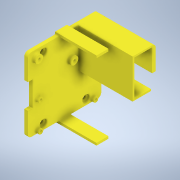
# Autodesk Inventor part: pieza_nasa
Saved by Autodesk Inventor 2021 (Build 250183000, 183)
## iProperties
Created: 2024-10-05
Part Number: pieza_nasa
Material: Generic
Document SubType Name: Modeling
Designer: hojan
Density: 1 g/cm^3
Appearance: Default
Author: hojan
Autodesk Inventor part; units mm, degrees
ref_plane "YZ Plane" through (0, 0, 0) normal (1, 0, 0) x (0, 1, 0)
ref_plane "XZ Plane" through (0, 0, 0) normal (0, 1, 0) x (-1, 0, 0)
ref_plane "XY Plane" through (0, 0, 0) normal (0, 0, 1) x (1, 0, 0)
sketch "Boceto1" plane through (0, 0, 0) normal (1, 0, 0) x (0, 1, 0)
  line L0 (-31, 31) -> (31, 31)
  line L1 (31, 31) -> (31, -31)
  line L2 (31, -31) -> (-31, -31)
  line L3 (-31, -31) -> (-31, 31)
  line L4 (-31, 31) -> (31, -31) construction
  line L5 (31, 31) -> (-31, -31) construction
  point P0 (0, 0)
  dimension "d0" = 62
  dimension "d1" = 62
  constraints: 12 end point, 2 midpoint, 2 parallel, 1 horizontal, 1 perpendicular
  measures "d0" distance of L1.end L2.end
  measures "d1" distance of L0.end L1.end
extrude "Extrusión1" add sketch "Boceto1" along normal blind 3
sketch "Boceto2" plane through (3, 0, 0) normal (1, 0, 0) x (0, 0, -1)
  line L0 (0, 0) -> (18, 0)
  line L1 (18, 0) -> (18, 26)
  line L2 (18, 26) -> (-18, 26)
  line L3 (-18, 26) -> (-18, -26)
  line L4 (-18, -26) -> (18, -26)
  circle A0 centre (-18, 26) radius 1.5
  circle A1 centre (18, 26) radius 1.5
  circle A2 centre (-18, -26) radius 1.5
  circle A3 centre (18, -26) radius 1.5
  dimension "d4" = 18
  dimension "d5" = 26
  dimension "d6" = 36
  dimension "d7" = 52
  dimension "d8" = 3
  dimension "d9" = 3
  dimension "d10" = 3
  dimension "d11" = 3
  constraints: 10 end point, 4 centre point, 4 coincident, 3 perpendicular, 1 horizontal, 1 point on line, 1 vertical
  measures "d4" distance of L0.start L0.end
  measures "d5" distance of L0.end L1.end
  measures "d6" distance of L1.end L2.end
  measures "d7" distance of L2.end L3.end
  measures "d8" diameter of A0
  measures "d9" diameter of A1
  measures "d10" diameter of A2
  measures "d11" diameter of A3
extrude "Extrusión2" cut sketch "Boceto2" against normal blind 3
fillet "Empalme1" radius 3 4 edges at (1.5, 31, 31) (1.5, 31, -31) (1.5, -31, 31) (1.5, -31, -31)
sketch "Boceto3" plane through (3, 0, 0) normal (1, 0, 0) x (0, 0, -1)
  circle A0 centre (-18, 26) radius 1.5 projected
  circle A1 centre (-18, 26) radius 3
  circle A2 centre (18, 26) radius 1.5 projected
  circle A3 centre (18, 26) radius 3
  circle A4 centre (18, -26) radius 1.5 projected
  circle A5 centre (18, -26) radius 3
  circle A6 centre (-18, -26) radius 1.5 projected
  circle A7 centre (-18, -26) radius 3
  point P0 (0, 0)
  dimension "d15" = 6
  dimension "d16" = 6
  dimension "d17" = 6
  dimension "d18" = 6
  constraints: 4 centre point, 4 coincident
  measures "d15" diameter of A1
  measures "d16" diameter of A3
  measures "d17" diameter of A5
  measures "d18" diameter of A7
extrude "Extrusión3" cut sketch "Boceto3" against normal blind 1.5 contours A0 | A1 | A2 | A3 | A5 | A7
sketch "Boceto4" plane through (3, 0, 0) normal (1, 0, 0) x (0, 0, -1)
  line L0 (0, 0) -> (-27, 0)
  line L1 (0, 0) -> (-31, 0)
  line L2 (-31, 28) -> (-31, -28) projected
  line L3 (-27, 0) -> (-27, 10.5)
  line L4 (-27, 10.5) -> (-31, 10.5)
  line L5 (-31, 10.5) -> (-31, -10.5)
  line L6 (-31, -10.5) -> (-27, -10.5)
  line L7 (-27, -10.5) -> (-27, 0)
  line L8 (0, 12.3803) -> (0, 8.7582)
  line L9 (27, 0) -> (27, 10.5)
  line L10 (27, 10.5) -> (31, 10.5)
  line L11 (31, 10.5) -> (31, -10.5)
  line L12 (31, -10.5) -> (27, -10.5)
  line L13 (27, -10.5) -> (27, 0)
  point P0 (31, 0)
  dimension "d21" = 27
  dimension "d22" = 31
  dimension "d23" = 10.5
  dimension "d24" = 21
  constraints: 26 end point, 6 symmetric about line, 5 perpendicular, 2 point on line, 2 vertical, 1 horizontal
  measures "d21" distance of L0.start L0.end
  measures "d22" distance of L0.start L1.end
  measures "d23" distance of L0.end L3.end
  measures "d24" distance of L4.end L5.end
extrude "Extrusión4" cut sketch "Boceto4" against normal blind 3
sketch "Boceto5" plane through (3, 0, 0) normal (1, 0, 0) x (0, 0, -1)
  arc A0 (-28, 31) -> (-31, 28) centre (-28, 28) ccw projected
  line L0 (-28, 28) -> (15, 28)
  line L1 (15, 28) -> (15, 7)
  line L2 (15, 7) -> (-28, 7)
  line L3 (-28, 28) -> (-28, 25.46)
  line L4 (-28, 25.46) -> (-21.4, 25.46)
  line L5 (15, 7) -> (15, 9.5)
  line L6 (15, 9.5) -> (8.4, 9.5)
  circle A1 centre (-21.4, 25.46) radius 1
  circle A2 centre (8.4, 9.5) radius 1
  circle A3 centre (-21.4, 25.46) radius 3.25
  circle A4 centre (8.4, 9.5) radius 3.25
  circle A5 centre (-18, 26) radius 1.5 projected
  circle A6 centre (-18, 26) radius 3 projected
  line L7 (-28, 28) -> (-31, 28)
  line L8 (-31, 28) -> (12, 28)
  line L9 (12, 7) -> (-31, 7)
  circle A7 centre (5.4, 9.5) radius 1
  line L10 (12, 28) -> (12, 7)
  circle A8 centre (5.4, 9.5) radius 3.25
  line L11 (12, 9.5) -> (5.4, 9.5)
  line L12 (12, 7) -> (12, 9.5)
  circle A9 centre (-24.4, 25.46) radius 1
  line L13 (-31, 25.46) -> (-24.4, 25.46)
  line L14 (-31, 28) -> (-31, 25.46)
  line L15 (-31, 28) -> (-34, 28)
  circle A10 centre (-24.4, 25.46) radius 3.25
  point P0 (0, 0)
  point P1 (-19.0678, 23.1965)
  point P2 (-19.8839, 28.3347)
  point P3 (-21, 26)
  point P4 (-21, 26)
  point P5 (-31, 31)
  dimension "d27" = 43
  dimension "d28" = 21
  dimension "d29" = 2.54
  dimension "d30" = 6.6
  dimension "d31" = 2.5
  dimension "d32" = 6.6
  dimension "d33" = 2
  dimension "d34" = 2
  dimension "d35" = 6.5
  dimension "d36" = 6.5
  dimension "d65" = 3
  dimension "d68" = 3
  constraints: 32 end point, 8 centre point, 8 coincident, 4 horizontal, 3 perpendicular, 2 point on line, 1 collinear, 1 vertical, 27 other
  measures "d27" distance of L0.start L0.end
  measures "d28" distance of L0.end L1.end
  measures "d29" distance of L0.start L3.end
  measures "d30" distance of L3.end L4.end
  measures "d31" distance of L1.end L5.end
  measures "d32" distance of L5.end L6.end
  measures "d33" diameter of A1
  measures "d34" diameter of A2
  measures "d35" diameter of A3
  measures "d36" diameter of A4
  measures "d65" distance of L0.start L7.end
  measures "d68" distance of L0.start L8.start
extrude "Extrusión5" add sketch "Boceto5" along normal blind 3 contours A10 L0 A3 | A3 L0 A10 | A8 A2 L11 A7 A4 | A4 A7 L2 A8 | A10 A1 L4 A9 A3 L0 | A10 L4 A9 A3 | A3 A9 L4 A1 A10 | A3 A9 L4 A10 L0 | A8 A2 L11 L6 | L6 L11 A2 A8 | A8 L2 A4 A7 L11 A2 | L2 A4 A8 | A8 A4 L2 | A10 A1 picked at (4.536, 6.8619) picked at (7.0312, 6.9529)
fillet "Empalme2" radius 1 2 edges at (3, 25.46, 27.65) (3, 9.5, -2.15)
sketch "Boceto6" plane through (3, 0, 0) normal (1, 0, 0) x (0, 0, -1)
  line L0 (-31, -35) -> (-31, -21.2021)
  line L1 (-31, 28) -> (-31, -28) projected
  line L2 (-31, -21.2021) -> (-23, -21.2021)
  line L3 (-23, -21.2021) -> (-23, 1.7979)
  line L4 (-23, 1.7979) -> (23.5, 1.7979)
  line L5 (23.5, 1.7979) -> (23.5, -21.2021)
  line L6 (23.5, -21.2021) -> (-23, -21.2021)
  line L7 (-1.735, -21.2021) -> (-1.735, -27.2021)
  circle A0 centre (23.5, 1.7979) radius 2
  circle A1 centre (23.5, -21.2021) radius 2
  circle A2 centre (-23, -21.2021) radius 2
  circle A3 centre (-23, 1.7979) radius 2
  circle A4 centre (-23, 1.7979) radius 1
  circle A5 centre (23.5, -21.2021) radius 1
  circle A6 centre (-23, -21.2021) radius 1
  circle A7 centre (23.5, 1.7979) radius 1
  line L8 (-23, -5.2021) -> (23.5, -5.2021)
  line L9 (23.5, -28.2021) -> (-23, -28.2021)
  line L10 (-1.735, -28.2021) -> (-1.735, -34.2021)
  circle A8 centre (-23, -5.2021) radius 1
  line L11 (-23, -28.2021) -> (-23, -5.2021)
  circle A9 centre (-23, -28.2021) radius 2
  circle A10 centre (-23, -5.2021) radius 2
  line L12 (23.5, -5.2021) -> (23.5, -28.2021)
  circle A11 centre (23.5, -28.2021) radius 1
  circle A12 centre (23.5, -5.2021) radius 1
  circle A13 centre (23.5, -28.2021) radius 2
  circle A14 centre (23.5, -5.2021) radius 2
  line L13 (-31, -28.2021) -> (-23, -28.2021)
  circle A15 centre (-23, -28.2021) radius 1
  point P0 (0, 0)
  point P1 (0, -7)
  point P2 (-31, -35)
  dimension "d40" = 23
  dimension "d41" = 46.5
  dimension "d42" = 8
  dimension "d43" = 13.7979
  dimension "d44" = 6
  dimension "d45" = 4
  dimension "d46" = 4
  dimension "d47" = 4
  dimension "d48" = 4
  dimension "d49" = 2
  dimension "d50" = 2
  dimension "d51" = 2
  dimension "d52" = 2
  dimension "d81" = 7
  constraints: 26 end point, 16 centre point, 16 coincident, 3 perpendicular, 3 point on line, 3 vertical, 1 collinear, 1 horizontal, 30 other
  measures "d40" distance of L2.end L3.end
  measures "d41" distance of L3.end L4.end
  measures "d42" distance of L0.end L2.end
  measures "d43" distance of L0.start L0.end
  measures "d44" distance of L7.start L7.end
  measures "d45" diameter of A0
  measures "d46" diameter of A1
  measures "d47" diameter of A2
  measures "d48" diameter of A3
  measures "d49" diameter of A4
  measures "d50" diameter of A5
  measures "d51" diameter of A6
  measures "d52" diameter of A7
  measures "d81" distance of point (0, 0) point (0, -7)
extrude "Extrusión6" add sketch "Boceto6" along normal up to surface (3 mm away) contours L13 A15 L9 A9 | A9 L11 A15 L13 | A9 L9 A15 L11 | A13 L12 A11 L9 | L9 A11 L12 A13 | A10 L3 A8 | L3 A8 L8 A10 | A10 L8 A8 L3 | A14 L5 A12 L8 | L8 A12 L5 A14 | A14 L5 A12
fillet "Empalme3" radius 1 4 edges at (3, -28.2021, -21.5) (3, -5.2021, -21.5) (3, -5.2021, 25) (3, -28.2021, 25)
sketch "Boceto8" plane through (3, 0, 0) normal (1, 0, 0) x (0, 0, -1)
  circle A0 centre (-23, -5.2021) radius 3 projected
  circle A1 centre (5.4, 9.5) radius 4.25 projected
  arc A2 (-20.6357, 27.4329) -> (-20.3583, 24.1457) centre (-24.4, 25.46) ccw projected
  arc A3 (-20.3583, 24.1457) -> (-20.6357, 27.4329) centre (-18, 26) ccw projected
  arc A4 (-20.9998, -25.9662) -> (-24.0825, -31) centre (-23, -28.2021) ccw projected
  arc A5 (-20.0002, -28.2359) -> (-20.9998, -25.9662) centre (-18, -26) ccw projected
  arc A6 (-21.9175, -31) -> (-20.0002, -28.2359) centre (-23, -28.2021) ccw projected
  line L0 (-21.9175, -31) -> (22.4175, -31) projected
  arc A7 (20.5736, -27.5416) -> (22.4175, -31) centre (23.5, -28.2021) ccw projected
  arc A8 (20.9264, -26.6606) -> (20.5736, -27.5416) centre (18, -26) ccw projected
  arc A9 (24.5825, -31) -> (20.9264, -26.6606) centre (23.5, -28.2021) ccw projected
  line L1 (24.5825, -31) -> (28, -31) projected
  arc A10 (28, -31) -> (31, -28) centre (28, -28) ccw projected
  line L2 (31, -28) -> (31, -10.5) projected
  line L3 (31, -10.5) -> (27, -10.5) projected
  line L4 (27, -10.5) -> (27, 10.5) projected
  line L5 (27, 10.5) -> (31, 10.5) projected
  line L6 (31, 10.5) -> (31, 28) projected
  arc A11 (31, 28) -> (28, 31) centre (28, 28) ccw projected
  line L7 (28, 31) -> (-28, 31) projected
  arc A12 (-28, 31) -> (-31, 28) centre (-28, 28) ccw projected
  line L8 (-31, 28) -> (-31, 10.5) projected
  line L9 (-31, 10.5) -> (-27, 10.5) projected
  line L10 (-27, 10.5) -> (-27, -10.5) projected
  line L11 (-27, -10.5) -> (-31, -10.5) projected
  line L12 (-31, -10.5) -> (-31, -28) projected
  arc A13 (-31, -28) -> (-28, -31) centre (-28, -28) ccw projected
  line L13 (-28, -31) -> (-24.0825, -31) projected
  circle A14 centre (18, 26) radius 3 projected
  circle A15 centre (23.5, -5.2021) radius 3 projected
  line L14 (28, 31) -> (-28, 31) projected
  line L15 (28, 31) -> (28, 29.5)
  line L16 (28, 29.5) -> (13, 29.5)
  line L17 (13, 29.5) -> (13, -0.5)
  line L18 (13, -0.5) -> (27, -0.5)
  line L19 (27, -10.5) -> (27, 10.5) projected
  line L20 (27, -0.5) -> (27, 10.5)
  line L21 (27, 10.5) -> (31, 10.5)
  line L22 (28, 29.5) -> (28, 10.5)
  line L23 (13, 29.5) -> (11.5, 29.5)
  line L24 (11.5, 29.5) -> (11.5, 31)
  line L25 (11.5, 29.5) -> (11.5, -2)
  line L26 (11.5, -2) -> (27, -2)
  line L27 (27, -2) -> (27, -0.5)
  point P0 (0, 0)
  dimension "d89" = 1.5
  dimension "d90" = 15
  dimension "d91" = 30
  dimension "d92" = 1.5
  dimension "d93" = 31.5
  constraints: 24 end point, 9 perpendicular, 5 point on line, 1 parallel, 1 vertical
  measures "d89" distance of L7.start L15.end
  measures "d90" distance of L15.end L16.end
  measures "d91" distance of L16.end L17.end
  measures "d92" distance of L16.end L23.end
  measures "d93" distance of L23.end L25.end
extrude "Extrusión8" add sketch "Boceto8" along normal blind 46 contours L7 L15 L16 L23 L24 | A11 L6 L5 L22 L15 | L23 L17 L18 L4 L26 L25
sketch "Boceto10" plane through (0, 0, 0) normal (-1, 0, 0) x (0, 0, 1)
  line L0 (28, -31) -> (-28, -31) projected
  line L1 (0, -31) -> (-5, -31)
  line L2 (-5, -31) -> (-5, -33)
  line L3 (-5, -33) -> (5, -33)
  line L4 (5, -33) -> (5, -31)
  line L5 (5, -31) -> (0, -31)
  line L6 (0, 0) -> (-3.9582, 0)
  line L7 (0, 31) -> (-5, 31)
  line L8 (-5, 31) -> (-5, 33)
  line L9 (-5, 33) -> (5, 33)
  line L10 (5, 33) -> (5, 31)
  line L11 (5, 31) -> (0, 31)
  dimension "d96" = 5
  dimension "d97" = 2
  dimension "d98" = 10
  constraints: 22 end point, 5 symmetric about line, 3 perpendicular, 2 point on line, 1 collinear, 1 horizontal, 1 midpoint
  measures "d96" distance of L1.start L1.end
  measures "d97" distance of L1.end L2.end
  measures "d98" distance of L2.end L3.end
extrude "Extrusión9" add sketch "Boceto10" against normal blind 35
fillet "Empalme6" radius 1 6 edges at (3, -31, 0) (3, 31, 0) (1.5, 31, 5) (1.5, 31, -5) (1.5, -31, 5) (1.5, -31, -5)
